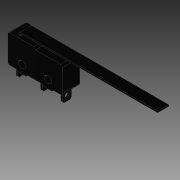
# Autodesk Inventor part: switch
Saved by Autodesk Inventor 2013 (Build 170138000, 138)
## iProperties
Created: 2013-05-08
Part Number: switch
Material: Acetal Resin, Black
Document SubType Name: Modeling
Designer: Administrator
Density: 1 g/cm^3
Author: Administrator
Autodesk Inventor part; units mm, degrees
ref_plane "YZ Plane" through (0, 0, 0) normal (1, 0, 0) x (0, 1, 0)
ref_plane "XZ Plane" through (0, 0, 0) normal (0, 1, 0) x (-1, 0, 0)
ref_plane "XY Plane" through (0, 0, 0) normal (0, 0, 1) x (1, 0, 0)
sketch "Sketch1" plane through (0, 0, 0) normal (0, 0, 1) x (1, 0, 0)
  line L0 (-6.8145, -6.5958) -> (-4.5145, -6.5958)
  line L1 (-4.5145, -6.5958) -> (-3.8195, -7.1258)
  line L2 (-3.8195, -7.1258) -> (-0.9895, -7.1258)
  line L3 (-0.9895, -7.1258) -> (-0.2945, -6.5958)
  line L4 (-0.2945, -6.5958) -> (4.8955, -6.5958)
  line L5 (4.8955, -6.5958) -> (5.5905, -7.1258)
  line L6 (5.5905, -7.1258) -> (8.4205, -7.1258)
  line L7 (8.4205, -7.1258) -> (9.1155, -6.5958)
  line L8 (9.1155, -6.5958) -> (11.5455, -6.5958)
  line L9 (12.2455, -5.8958) -> (12.2455, 2.1742)
  line L10 (11.5455, 2.8742) -> (2.5355, 2.8742)
  line L11 (-7.5145, 2.8542) -> (-7.5145, -5.8958)
  line L12 (-2.4045, -0.6574) -> (-2.4045, -6.9746)
  line L13 (7.0055, -0.6574) -> (7.0055, -6.9746)
  line L14 (-8.0311, -4.1558) -> (13.5632, -4.1558)
  circle A0 centre (-2.4045, -4.1558) radius 1.25
  circle A1 centre (7.0055, -4.1558) radius 1.25
  line L15 (1.9155, 3.5542) -> (2.5355, 2.8742)
  line L16 (-4.4145, 3.5542) -> (-4.4145, 4.2242)
  line L17 (-3.9145, 4.7242) -> (45.5855, 4.7242)
  line L18 (45.5855, 4.7242) -> (45.5855, 4.2442)
  line L19 (45.5855, 4.2442) -> (-3.4345, 4.2442)
  line L20 (-3.9345, 3.7442) -> (-3.9345, 3.5542)
  line L21 (-6.8145, 3.5542) -> (-4.4145, 3.5542)
  line L22 (-3.9345, 3.5542) -> (1.9155, 3.5542)
  arc A2 (-6.8145, 3.5542) -> (-7.5145, 2.8542) centre (-6.8145, 2.8542) ccw
  arc A3 (-7.5145, -5.8958) -> (-6.8145, -6.5958) centre (-6.8145, -5.8958) ccw
  arc A4 (11.5455, -6.5958) -> (12.2455, -5.8958) centre (11.5455, -5.8958) ccw
  arc A5 (12.2455, 2.1742) -> (11.5455, 2.8742) centre (11.5455, 2.1742) ccw
  arc A6 (-3.9145, 4.7242) -> (-4.4145, 4.2242) centre (-3.9145, 4.2242) ccw
  arc A7 (-3.4345, 4.2442) -> (-3.9345, 3.7442) centre (-3.4345, 3.7442) ccw
  point P0 (-7.5145, -6.5958)
  point P1 (12.2455, 2.8742)
  point P2 (-7.5145, 3.5542)
  point P3 (-4.4145, 4.7242)
  dimension "d21" = 2.5
  dimension "d22" = 2.5
  dimension "d23" = 2.97
  dimension "d24" = 0.53
  dimension "d25" = 2.83
  dimension "d26" = 3
  dimension "d27" = 5.11
  dimension "d28" = 9.41
  dimension "d29" = 19.76
  dimension "d31" = 9.47
  dimension "d32" = 9.71
  dimension "d33" = 9.43
  dimension "d40" = 10.15
  dimension "d41" = 3.1
  dimension "d42" = 0.48
  dimension "d43" = 0.48
  dimension "d44" = 1.17
  dimension "d45" = 50
  dimension "d46" = 0.7
  dimension "d47" = 0.5
  constraints: 46 end point, 12 point on circle, 12 point on line, 12 tangent, 11 parallel, 8 centre point, 7 collinear, 5 perpendicular, 4 equal radius, 1 horizontal, 2 other
  measures "d21" diameter of A0
  measures "d22" diameter of A1
  measures "d23" distance from line of A0.centre L2
  measures "d24" distance between parallel lines of L0 L2
  measures "d25" distance of L1.end L2.end
  measures "d26" distance of point (-7.515, -6.596) L0.end
  measures "d27" distance between parallel lines of L11 L12
  measures "d28" distance of A1.centre A0.centre
  measures "d29" distance between parallel lines of L9 L11
  measures "d31" distance between parallel lines of L8 L10
  measures "d32" distance of point (12.245, 2.874) L10.end
  measures "d33" distance of point (-7.515, 3.554) L15.start
  measures "d40" distance of point (-7.515, 3.554) point (-7.515, -6.596)
  measures "d41" distance between parallel lines of L11 L16
  measures "d42" distance between parallel lines of L16 L20
  measures "d43" distance between parallel lines of L17 L19
  measures "d44" distance between parallel lines of L22 L17
  measures "d45" distance of point (-4.415, 4.724) L17.end
  measures "d46" radius of A2
  measures "d47" radius of A6
extrude "Extrusion1" add sketch "Sketch1" along normal blind 6.26 contours A3 L11 L14 A0 A1 L9 A4 L8 L7 L6 L5 L4 L3 L2 L1 L0 | L11 A2 L21 L16 A6 L17 L18 L19 A7 L20 L22 L15 L10 A5 L9 L14 A1 A0
sketch "Sketch2" plane through (0, 0, 6.26) normal (0, 0, 1) x (1, 0, 0)
  line L0 (-3.9345, 3.5542) -> (-3.9345, 3.7442) projected
  arc A0 (-3.4345, 4.2442) -> (-3.9345, 3.7442) centre (-3.4345, 3.7442) ccw projected
  line L1 (-3.4345, 4.2442) -> (45.5855, 4.2442) projected
  line L2 (45.5855, 4.2442) -> (45.5855, 4.7242) projected
  line L3 (45.5855, 4.7242) -> (-3.9145, 4.7242) projected
  arc A1 (-3.9145, 4.7242) -> (-4.4145, 4.2242) centre (-3.9145, 4.2242) ccw projected
  line L4 (-4.4145, 4.2242) -> (-4.4145, 3.5542) projected
  line L5 (-7.5145, 2.8542) -> (-7.5145, -5.8958) projected
  line L6 (-4.4145, 3.5542) -> (-3.9345, 3.5542)
  point P0 (0, 0)
  constraints: 2 end point, 1 perpendicular
extrude "Extrusion2" cut sketch "Sketch2" against normal blind 0.96
sketch "Sketch3" plane through (0, 0, 0) normal (0, 0, -1) x (-1, 0, 0)
  line L0 (4.4145, 3.5542) -> (4.4145, 4.2242) projected
  arc A0 (4.4145, 4.2242) -> (3.9145, 4.7242) centre (3.9145, 4.2242) ccw projected
  line L1 (3.9145, 4.7242) -> (-45.5855, 4.7242) projected
  line L2 (-45.5855, 4.7242) -> (-45.5855, 4.2442) projected
  line L3 (-45.5855, 4.2442) -> (3.4345, 4.2442) projected
  arc A1 (3.9345, 3.7442) -> (3.4345, 4.2442) centre (3.4345, 3.7442) ccw projected
  line L4 (3.9345, 3.7442) -> (3.9345, 3.5542) projected
  line L5 (0.9895, -7.1258) -> (3.8195, -7.1258) projected
  line L6 (3.9345, 3.5542) -> (4.4145, 3.5542)
  point P0 (0, 0)
  constraints: 2 end point, 1 parallel
extrude "Extrusion3" cut sketch "Sketch3" against normal blind 1.22
sketch "Sketch4" plane through (-0.2945, -6.5958, 0) normal (0, -1, 0) x (1, 0, 0)
  line L0 (3.09, 4.71) -> (3.67, 4.71)
  line L1 (3.67, 4.71) -> (3.67, 1.43)
  line L2 (3.67, 1.43) -> (3.09, 1.43)
  line L3 (3.09, 1.43) -> (3.09, 4.71)
  line L4 (-5.74, 4.71) -> (-5.16, 4.71)
  line L5 (-5.16, 4.71) -> (-5.16, 1.43)
  line L6 (-5.16, 1.43) -> (-5.74, 1.43)
  line L7 (-5.74, 1.43) -> (-5.74, 4.71)
  line L8 (10.38, 4.71) -> (10.96, 4.71)
  line L9 (10.96, 4.71) -> (10.96, 1.43)
  line L10 (10.96, 1.43) -> (10.38, 1.43)
  line L11 (10.38, 1.43) -> (10.38, 4.71)
  line L12 (-6.52, 6.26) -> (-4.22, 6.26) projected
  line L13 (-7.22, 0) -> (-7.22, 6.26) projected
  point P0 (0.2945, 0)
  dimension "d52" = 3.28
  dimension "d54" = 0.58
  dimension "d55" = 1.55
  dimension "d56" = 1.48
  dimension "d57" = 9.41
  dimension "d58" = 7.87
  constraints: 24 end point, 6 parallel, 4 equal length, 3 horizontal, 3 perpendicular, 2 collinear
  measures "d52" distance of L0.end L1.end
  measures "d54" distance of L0.start L0.end
  measures "d55" distance between parallel lines of L12 L4
  measures "d56" distance between parallel lines of L13 L7
  measures "d57" distance between parallel lines of L1 L7
  measures "d58" distance between parallel lines of L9 L3
extrude "Extrusion4" add sketch "Sketch4" along normal blind 4.11
sketch "Sketch5" plane through (-6.0345, -10.7058, 1.43) normal (-1, 0, 0) x (0, 0, 1)
  line L0 (0, 4.11) -> (0, 0) projected
  line L1 (3.28, 0) -> (0, 0) projected
  line L2 (3.28, 4.11) -> (3.28, 0) projected
  circle A0 centre (1.64, 1.86) radius 0.77
  line L3 (0, 0.5657) -> (0.5657, 0)
  line L4 (0, 0.5657) -> (0.8, 0.5657) construction
  line L5 (2.7143, 0) -> (3.28, 0.5657)
  point P0 (-1.43, 10.7058)
  dimension "d61" = 1.54
  dimension "d62" = 1.86
  dimension "d63" = 3.28
  dimension "d64" = 1.64
  dimension "d65" = 45
  dimension "d66" = 0.8
  constraints: 6 end point, 4 point on line, 2 equal length, 1 centre point, 1 horizontal, 1 perpendicular
  measures "d61" diameter of A0
  measures "d62" distance from line of L1 A0.centre
  measures "d63" distance of L1.start L0.end
  measures "d64" distance from line of L2 A0.centre
  measures "d65" angle of L3 L4
  measures "d66" distance of L3.start L3.end
extrude "Extrusion5" cut sketch "Sketch5" against normal through all
equation "\"d22\" = d21"
equation "\"d43\" = d42"
equation "\"d64\" = 0.5 * d63"
equation "\"d7\" = d6"
equation "\"d6\" = 2.9"
body "Solid1"
